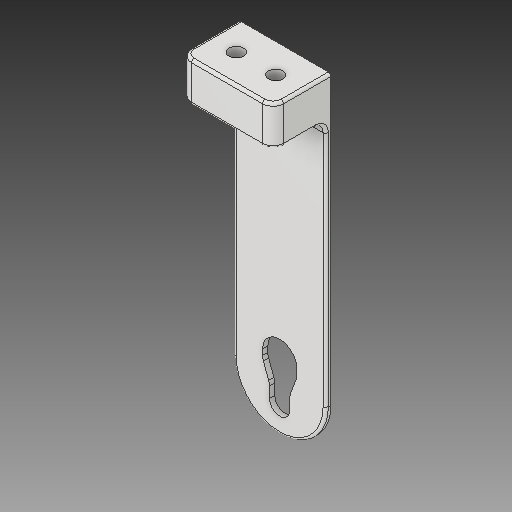
# Autodesk Inventor part: Bras
Saved by Autodesk Inventor 2017 (Build 210142000, 142)
## iProperties
Company: FABLAB Frenchmakers
Part Number: Bras
Project: 1400-PopCorn Machine
Material: Plastique ABS
Catalog Web Link: http://www.frenchmakers.com/
Document SubType Name: Modeling
Designer: FABLAB Frenchmakers
Density: 1.06 g/cm^3
Appearance: Lisse - Blanc
Stock Number: 1400-08-01
Mass: 18.2792 g
Surface Area: 111.625 cm^2
Volume: 17.2445 cm^3
Author: Adrien MARY
Autodesk Inventor part; units mm, degrees
ref_plane "YZ Plane" through (0, 0, 0) normal (1, 0, 0) x (0, 1, 0)
ref_plane "XZ Plane" through (0, 0, 0) normal (0, 1, 0) x (-1, 0, 0)
ref_plane "XY Plane" through (0, 0, 0) normal (0, 0, 1) x (1, 0, 0)
sketch "Esquisse1" plane through (0, 0, 0) normal (0, 0, 1) x (1, 0, 0)
  line L0 (17.5, -109.2) -> (17.5, 0)
  line L1 (17.5, 0) -> (-17.5, 0)
  line L2 (-17.5, 0) -> (-17.5, -109.2)
  arc A0 (-17.5, -109.2) -> (17.5, -109.2) centre (0, -109.2) ccw
  arc A1 (-3.875, -116.7) -> (3.875, -116.7) centre (0, -116.7) ccw
  arc A2 (6.5, -101.7) -> (-6.5, -101.7) centre (0, -101.7) ccw
  line L3 (-3.875, -111.7) -> (-3.875, -116.7)
  line L4 (3.875, -116.7) -> (3.875, -111.7)
  line L5 (-6.5, -101.7) -> (-6.5, -104.7)
  line L6 (-6.5, -104.7) -> (-3.875, -111.7)
  line L7 (3.875, -111.7) -> (6.5, -104.7)
  line L8 (6.5, -104.7) -> (6.5, -101.7)
  point P0 (0, 0)
  point P1 (0, 0)
  dimension "d0" = 35
  dimension "d1" = 126.7
  dimension "d3" = 3
  dimension "d4" = 6.5
  dimension "d5" = 5
  dimension "d6" = 15
  dimension "d7" = 116.7
  dimension "d8" = 3.875
  constraints: 18 end point, 6 point on circle, 6 tangent, 4 vertical, 3 centre point, 2 equal length, 2 horizontal alignment, 2 parallel, 2 vertical alignment, 1 coincident, 1 horizontal, 1 midpoint
  measures "d0" distance of L0.end L1.end
  measures "d3" distance of L5.start L5.end
  measures "d4" radius of A2
  measures "d5" distance of L3.start L3.end
  measures "d6" distance of A1.centre A2.centre
  measures "d7" distance from line of L1 A1.centre
  measures "d8" radius of A1
extrude "Embase" add sketch "Esquisse1" along normal blind 2
sketch "Esquisse2" plane through (0, 0, 2) normal (0, 0, 1) x (1, 0, 0)
  line L0 (-17.5, -15) -> (17.5, -15)
  line L1 (17.5, -15) -> (17.5, 0)
  line L2 (17.5, 0) -> (-17.5, 0)
  line L3 (-17.5, 0) -> (-17.5, -15)
  line L4 (17.5, 0) -> (-17.5, 0) projected
  line L5 (-17.5, 0) -> (-17.5, -109.2) projected
  line L6 (17.5, -109.2) -> (17.5, 0) projected
  point P0 (0, 0)
  dimension "d11" = 15
  constraints: 8 end point, 3 collinear, 2 parallel, 1 horizontal, 1 perpendicular
  measures "d11" distance of L1.end L0.end
extrude "Support" add sketch "Esquisse2" along normal blind 20
sketch "Esquisse3" plane through (-17.5, -15, 2) normal (0, -1, 0) x (1, 0, 0)
  line L0 (0, -2) -> (0, 20) projected
  point P0 (17.5, -2)
  point P1 (10, 9)
  point P2 (25, 9)
  point P3 (0, 9)
  dimension "Entraxe" = 15
  dimension "d15" = 7.5
  constraints: 2 horizontal alignment, 1 midpoint
  measures "Entraxe" distance of point (25, 9) point (10, 9)
  measures "d15" horizontal distance of point (17.5, -2) point (10, 9)
hole "Passage vis" at (-7.5, -15, 11) at (7.5, -15, 11) direction (0, 1, 0) diameter 5.5 end through all counterbore diameter 10 counterbore depth 5.5 clearance for "Vis d'assemblage à tête hexagonale ISO 24017" size "M5" standard "ISO"
fillet "Congé1" radius 4 3 edges at (-17.5, -7.5, 22) (17.5, -7.5, 22) (0, -15, 2)
fillet "Congé1" radius 5 4 edges at (3.875, -111.7, 1) (6.5, -104.7, 1) (-6.5, -104.7, 1) (-3.875, -111.7, 1)
fillet "Congé2" radius 1 15 edges at (16.3286, -15, 20.8286) (17.5, -15, 12) (17.5, -16.1714, 3.1714) (17.5, -64.0997, 2) (0, -126.7, 2) (-17.5, -64.0998, 2) (-17.5, -16.1714, 3.1714) (-17.5, -15, 12) (-16.3286, -15, 20.8286) (0, -15, 22) (-16.3286, 0, 20.8286) (-17.5, 0, 9.0003) (16.3286, 0, 20.8286) (17.5, 0, 9.0003) (0, 0, 22)
equation "\"d15\" = 0.5 * Entraxe"
